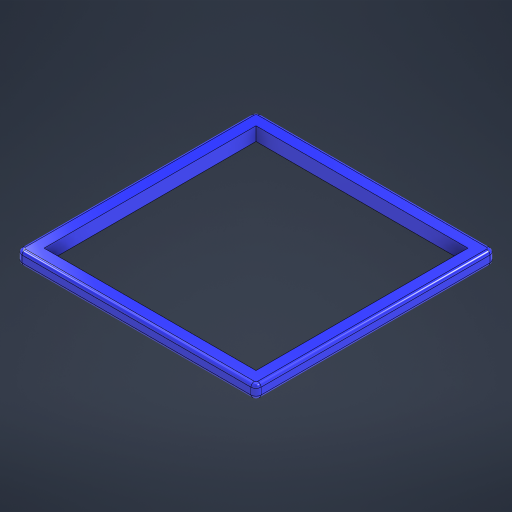
# Autodesk Inventor part: 200555
Saved by Autodesk Inventor 2023.1 (Build 271208000, 208)
## iProperties
Created: 2023-01-06
Part Number: 200555
Material: Generic
Document SubType Name: Modeling
Designer: Byron Robotics
Mass: 8457.66 g
Surface Area: 6453.35 cm^2
Volume: 8457.66 cm^3
Density: 1 g/cm^3
Appearance: Blue - Wall Paint - Glossy
Author: Byron Robotics
Autodesk Inventor part; units mm, degrees
ref_plane "YZ Plane" through (0, 0, 0) normal (1, 0, 0) x (0, 1, 0)
ref_plane "XZ Plane" through (0, 0, 0) normal (0, 1, 0) x (-1, 0, 0)
ref_plane "XY Plane" through (0, 0, 0) normal (0, 0, 1) x (1, 0, 0)
sketch "Sketch1" plane through (0, 0, 0) normal (0, 1, 0) x (-1, 0, 0)
  line L0 (0, 0) -> (793.75, 0)
  line L1 (793.75, 0) -> (793.75, 793.75)
  line L2 (793.75, 793.75) -> (0, 793.75)
  line L3 (0, 793.75) -> (0, 0)
  line L4 (0, 793.75) -> (793.75, 0) construction
  line L5 (793.75, 793.75) -> (0, 0) construction
  line L6 (844.55, -50.8) -> (-50.8, -50.8)
  line L7 (-50.8, -50.8) -> (-50.8, 844.55)
  line L8 (-50.8, 844.55) -> (844.55, 844.55)
  line L9 (844.55, 844.55) -> (844.55, -50.8)
  line L10 (844.55, -50.8) -> (-50.8, 844.55) construction
  line L11 (-50.8, -50.8) -> (844.55, 844.55) construction
  point P0 (396.875, 396.875)
  dimension "d0" = 793.75
  dimension "d1" = 50.8
  dimension "d2" = 50.8
  constraints: 24 end point, 4 parallel, 4 perpendicular, 3 midpoint, 2 horizontal
  measures "d0" distance of L1.end L2.end
  measures "d1" distance between parallel lines of L3 L7
  measures "d2" distance between parallel lines of L8 L2
extrude "Extrusion1" add sketch "Sketch1" along normal blind 50.8
fillet "Fillet1" radius 12.7 8 edges at (-396.875, 50.8, 844.55) (-844.55, 50.8, 396.875) (-396.875, 50.8, -50.8) (50.8, 50.8, 396.875) (-396.875, 0, 844.55) (50.8, 0, 396.875) (-396.875, 0, -50.8) (-844.55, 0, 396.875)
fillet "Fillet2" radius 19.05 12 edges at (47.0803, 47.0803, -47.0803) (47.0803, 3.7197, -47.0803) (50.8, 25.4, -50.8) (47.0803, 47.0803, 840.8303) (47.0803, 3.7197, 840.8303) (50.8, 25.4, 844.55) (-840.8303, 47.0803, 840.8303) (-840.8303, 3.7197, 840.8303) (-844.55, 25.4, 844.55) (-840.8303, 47.0803, -47.0803) (-840.8303, 3.7197, -47.0803) (-844.55, 25.4, -50.8)
body "Solid1"
